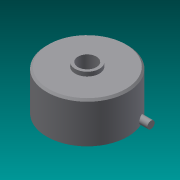
# Autodesk Inventor part: meh-30-pエンコーダ
Saved by Autodesk Inventor 2015 (Build 190159000, 159)
## iProperties
Created: 2016-02-18
Part Number: meh-30-pエンコーダ
Material: 一般
Document SubType Name: Modeling
Designer: buzztaka
Density: 1 g/cm^3
Appearance: 既定
Author: buzztaka
Autodesk Inventor part; units mm, degrees
ref_plane "YZ Plane" through (0, 0, 0) normal (1, 0, 0) x (0, 1, 0)
ref_plane "XZ Plane" through (0, 0, 0) normal (0, 1, 0) x (-1, 0, 0)
ref_plane "XY Plane" through (0, 0, 0) normal (0, 0, 1) x (1, 0, 0)
sketch "スケッチ1" plane through (0, 0, 0) normal (0, 0, 1) x (1, 0, 0)
  circle A0 centre (0, 0) radius 22
  dimension "d0" = 44
  constraints: 1 centre point, 1 coincident
  measures "d0" diameter of A0
extrude "押し出し1" add sketch "スケッチ1" along normal blind 22
chamfer "面取り1" distance 1 angle 45 1 edges at (-22, 0, 22)
sketch "スケッチ2" plane through (0, 0, 22) normal (0, 0, 1) x (1, 0, 0)
  circle A0 centre (0, 0) radius 6.6
  dimension "d6" = 13.2
  constraints: 1 centre point, 1 coincident
  measures "d6" diameter of A0
extrude "押し出し2" add sketch "スケッチ2" along normal blind 2.25
sketch "スケッチ6" plane through (0, 0, 0) normal (0, 0, 1) x (1, 0, 0)
  point P0 (0, 0)
sketch "スケッチ8" plane through (0, 0, 0) normal (0, 1, 0) x (-1, 0, 0)
  point P0 (0, 0)
sketch "スケッチ9" plane through (0, 0, 0) normal (1, 0, 0) x (0, 1, 0)
  line L0 (-22, 0) -> (22, 0) projected
  circle A0 centre (9.6776, 2.25) radius 2
  point P0 (0, 0)
  dimension "d30" = 2.25
  dimension "d31" = 4
  constraints: 1 centre point, 1 coincident
  measures "d30" distance from line of L0 point (9.678, 2.25)
  measures "d31" diameter of A0
extrude "押し出し3" add sketch "スケッチ9" along normal blind 25
sketch "スケッチ12" plane through (0, 0, 0) normal (0, 0, -1) x (-1, 0, 0)
  circle A0 centre (0, 0) radius 6
  dimension "d44" = 12
  constraints: 1 centre point, 1 coincident
  measures "d44" diameter of A0
extrude "押し出し5" add sketch "スケッチ12" along normal blind 0.75
sketch "スケッチ13" plane through (0, 0, 24.25) normal (0, 0, 1) x (1, 0, 0)
  point P0 (0, 0)
  point P1 (0, 0)
  constraints: 1 coincident
hole "穴4" at (0, 0, 24.25) direction (0, 0, -1) diameter 10 end through all
sketch "スケッチ14" plane through (0, 0, 0) normal (0, 0, -1) x (-1, 0, 0)
  point P0 (0, 0)
  point P1 (-18, 0)
  point P2 (9, -15.5885)
  point P3 (9, 15.5885)
  dimension "d54" = 18
  dimension "d57" = 360
  constraints: 4 other
  measures "d54" distance of point (0, 0) point (-18, 0)
hole "穴5" at (18, 0, 0) at (-9, -15.5885, 0) at (-9, 15.5885, 0) direction (0, 0, 1) diameter 3 depth 5 tip angle 118
